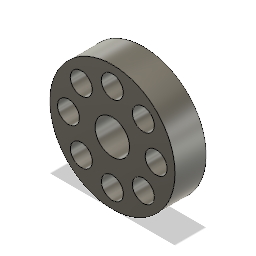
507d5d83-2fdb-473b-99c4-d262411869d8 (Autodesk Fusion 360 design; units mm, degrees)
Autodesk Fusion 360 part; units mm, degrees
sketch "Sketch1" plane through (0, 0, 0) normal (0, 0, 1) x (1, 0, 0)
  circle A0 centre (0, 0) radius 40
  circle A1 centre (0, 0) radius 28
  circle A2 centre (0, 0) radius 11
  circle A3 centre (28, 0.0227) radius 7
  circle A4 centre (19.7829, 19.815) radius 7
  circle A5 centre (-0.0227, 28) radius 7
  circle A6 centre (-19.815, 19.7829) radius 7
  circle A7 centre (-28, -0.0227) radius 7
  circle A8 centre (-19.7829, -19.815) radius 7
  circle A9 centre (0.0227, -28) radius 7
  circle A10 centre (19.815, -19.7829) radius 7
  dimension "d1" = 80
  dimension "d2" = 56
  dimension "d3" = 22
  dimension "d4" = 14
  dimension "d6" = 360
  measures "d1" diameter of A0
  measures "d2" diameter of A1
  measures "d3" diameter of A2
  measures "d4" diameter of A3
extrude "Extrude1" add sketch "Sketch1" along normal blind 20 contours A0 | A1 A3 A4 A5 A6 A7 A8 A9 A10
